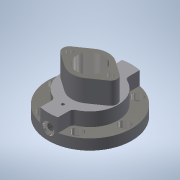
# Autodesk Inventor part: součást 5
Saved by Autodesk Inventor 2022 (Build 260153000, 153)
## iProperties
Created: 2009-01-29
Part Number: součást 5
Document SubType Name: Modeling
Designer: 27262
Material: Generic
Density: 1 g/cm^3
Appearance: Default
Mass: 444.242 g
Surface Area: 751.363 cm^2
Volume: 444.242 cm^3
Author: 27262
Autodesk Inventor part; units mm, degrees
note: some values were not read from the file. Chosen so that the rebuilt part matches the saved one: direction of "Hole3".
ref_plane "YZ Plane" through (0, 0, 0) normal (1, 0, 0) x (0, 1, 0)
ref_plane "XZ Plane" through (0, 0, 0) normal (0, 1, 0) x (-1, 0, 0)
sketch "Sketch1" plane through (0, 0, 0) normal (0, 0, 1) x (1, 0, 0)
  line L0 (-57, 0) -> (76, 0) projected
  line L1 (0, -85.2) -> (0, 113.6) projected
  line L2 (15, -69.3974) -> (15, -50.5099)
  line L3 (15, 50.5099) -> (15, 69.3974)
  arc A0 (15, 69.3974) -> (-15, 69.3974) centre (0, 0) ccw
  arc A1 (-15, -69.3974) -> (15, -69.3974) centre (0, 0) ccw
  line L4 (-15, -69.3974) -> (-15, -50.5099)
  line L5 (-15, 50.5099) -> (-15, 69.3974)
  arc A2 (-19.6847, 43.2292) -> (-19.6847, -43.2292) centre (0, 0) ccw
  arc A3 (19.6847, -43.2292) -> (19.6847, 43.2292) centre (0, 0) ccw
  arc A4 (-19.6847, 43.2292) -> (-15, 50.5099) centre (-23, 50.5099) ccw
  arc A5 (15, 50.5099) -> (19.6847, 43.2292) centre (23, 50.5099) ccw
  arc A6 (19.6847, -43.2292) -> (15, -50.5099) centre (23, -50.5099) ccw
  arc A7 (-15, -50.5099) -> (-19.6847, -43.2292) centre (-23, -50.5099) ccw
  dimension "d3" = 47.5
  dimension "d5" = 71
  dimension "d6" = 8
  dimension "d7" = 30
  constraints: 16 point on circle, 8 centre point, 8 end point, 8 tangent, 5 equal radius, 4 parallel, 2 collinear, 2 point on line, 1 coincident, 1 other
  measures "d3" radius of A2
  measures "d5" radius of A0
  measures "d6" radius of A4
  measures "d7" distance between parallel lines of L3 L5
extrude "Extrusion1" add sketch "Sketch1" along normal blind 41
sketch "Sketch2" plane through (0, 0, 0) normal (0, 0, 1) x (1, 0, 0)
  arc A0 (-15, -69.3974) -> (15, -69.3974) centre (0, 0) ccw projected
  circle A1 centre (0, 0) radius 71
  constraints: 1 coincident, 3 other
extrude "Extrusion2" add sketch "Sketch2" along normal blind 18
sketch "Sketch3" plane through (0, 0, 41) normal (0, 0, 1) x (1, 0, 0)
  arc A0 (-19.6847, 43.2292) -> (-19.6847, -43.2292) centre (0, 0) ccw projected
  line L0 (-57, 0) -> (76, 0) projected
  line L1 (0, -85.2) -> (0, 113.6) projected
  arc A1 (-41.2857, 9.0272) -> (-41.2857, -9.0272) centre (-35, 0) ccw
  line L2 (-41.2857, 9.0272) -> (-17.7143, 25.4402)
  line L3 (-41.2857, -9.0272) -> (-17.7143, -25.4402)
  arc A2 (41.2857, -9.0272) -> (41.2857, 9.0272) centre (35, 0) ccw
  line L4 (41.2857, 9.0272) -> (17.7143, 25.4402)
  line L5 (41.2857, -9.0272) -> (17.7143, -25.4402)
  arc A3 (-17.7143, -25.4402) -> (17.7143, -25.4402) centre (0, 0) ccw
  arc A4 (17.7143, 25.4402) -> (-17.7143, 25.4402) centre (0, 0) ccw
  dimension "d15" = 11
  dimension "d17" = 31
  dimension "d18" = 70
  constraints: 8 end point, 8 point on circle, 5 symmetric about line, 4 centre point, 4 tangent, 1 coincident, 1 concentric, 1 point on line, 1 other
  measures "d15" radius of A1
  measures "d17" radius of A4
  measures "d18" distance of A2.centre A1.centre
extrude "Extrusion3" add sketch "Sketch3" along normal blind 37
sketch "Sketch4" plane through (0, 0, 78) normal (0, 0, 1) x (1, 0, 0)
  arc A0 (-41.2857, 9.0272) -> (-41.2857, -9.0272) centre (-35, 0) ccw projected
  arc A1 (41.2857, -9.0272) -> (41.2857, 9.0272) centre (35, 0) ccw projected
  constraints: 2 coincident
hole "Hole1" at (-35, 0, 78) at (35, 0, 78) direction (0, 0, -1) diameter 10 depth 15 tip angle 118
sketch "Sketch5" plane through (0, 0, 0) normal (0, 1, 0) x (-1, 0, 0)
  line L0 (0, -7.8) -> (0, 101.4) projected
  line L1 (-17.7143, 78) -> (17.7143, 78) projected
  line L2 (0, 78) -> (23, 78)
  line L3 (23, 78) -> (23, 41)
  line L4 (23, 41) -> (15, 41)
  line L5 (0, 0) -> (0, 78)
  line L6 (15, 41) -> (15, 32)
  line L7 (15, 32) -> (18.1794, 32)
  line L8 (22.0431, 29.0353) -> (25, 18)
  line L9 (25, 18) -> (31, 18)
  line L10 (31, 18) -> (31, 0)
  line L11 (-71, 0) -> (71, 0) projected
  arc A0 (22.0431, 29.0353) -> (18.1794, 32) centre (18.1794, 28) ccw
  point P0 (21.2487, 32)
  dimension "d28" = 15
  dimension "d29" = 46
  dimension "d30" = 62
  dimension "d31" = 30
  dimension "d32" = 50
  dimension "d33" = 37
  dimension "d34" = 18
  dimension "d35" = 14
  dimension "d36" = 4
  constraints: 18 end point, 4 parallel, 3 point on line, 2 midpoint, 2 perpendicular, 2 point on circle, 2 tangent, 1 centre point, 1 horizontal
  measures "d28" angle of L10 L8
  measures "d29" diameter of L3 L0
  measures "d30" diameter of L10 L0
  measures "d31" diameter of L6 L0
  measures "d32" diameter of L8.end L0
  measures "d33" distance of L2.end L3.end
  measures "d34" distance of L9.end L10.end
  measures "d35" vertical distance of point (21.249, 32) L8.end
  measures "d36" radius of A0
revolve "Revolution1" cut sketch "Sketch5" angle 360 about axis through (0, 0, -10) along (0, 0, 1)
sketch "Sketch6" plane through (0, 0, 0) normal (1, 0, 0) x (0, 1, 0)
  line L0 (31, 18) -> (-31, 18) projected
  line L1 (-71, 18) -> (0, 18)
  line L2 (0, -4.1) -> (0, 53.3) projected
  line L3 (-81.2, 0) -> (61.6, 0) projected
  line L4 (-71, 0) -> (-71, 41) projected
  line L5 (-67, 20.5) -> (-67, 28)
  line L6 (-67, 28) -> (-71, 28)
  line L7 (-71, 28) -> (-71, 18)
  line L8 (-71, 18) -> (0, 18)
  line L9 (0, 18) -> (0, 20.5)
  line L10 (0, 20.5) -> (-67, 20.5)
  dimension "d38" = 4
  dimension "d39" = 20
  dimension "d40" = 5
  constraints: 14 end point, 3 point on line, 2 collinear, 2 parallel, 1 horizontal, 1 perpendicular
  measures "d38" distance of L5.end L6.end
  measures "d39" diameter of L6 L1
  measures "d40" diameter of L10 L1
revolve "Revolution2" cut sketch "Sketch6" angle 360 about axis through (0, -71, 18) along (0, 1, 0) contours L0 L1 L4 L6 L5 L10 L2
hole "Hole2" at (0, -67, 18) direction (0, 1, 0) diameter 11.445 depth 28 tip angle 118 thread size "G13.157x1.337" designation "G 1/4" standard "JIS Pipe Threads"
sketch "Sketch7" plane through (0, 0, 41) normal (0, 0, 1) x (1, 0, 0)
  arc A0 (-17.7143, -25.4402) -> (17.7143, -25.4402) centre (0, 0) ccw projected
  line L0 (0, -85.2) -> (0, 113.6) projected
  arc A1 (19.6847, -43.2292) -> (19.6847, 43.2292) centre (0, 0) ccw projected
  arc A2 (19.6847, -43.2292) -> (19.6847, 43.2292) centre (0, 0) ccw projected
  point P0 (0, -46)
  dimension "d52" = 46
  constraints: 1 point on line
  measures "d52" distance of A0.centre point (0, -46)
hole "Hole3" at (0, -46, 41) direction (0, 0, -1) diameter 5 end up to surface
ref_plane "Work Plane1" through (0, 0, 0) normal (0, 1, 0) x (-1, 0, 0)
sketch "Sketch8" plane through (0, 0, 18) normal (0, 0, 1) x (1, 0, 0)
  arc A0 (-15, 69.3974) -> (-15, -69.3974) centre (0, 0) ccw projected
  line L0 (-85.2, 0) -> (113.6, 0) projected
  point P0 (59, 0)
  dimension "d61" = 59
  constraints: 1 point on line
  measures "d61" distance of A0.centre point (59, 0)
hole "Hole4" at (59, 0, 18) direction (0, 0, -1) diameter 11 end through all counterbore diameter 18 counterbore depth 11
pattern_circular "Circular Pattern1" count 6 over 360 about axis through (0, 0, 0) along (0, 0, 1) of "Hole4"
body "Solid1"
